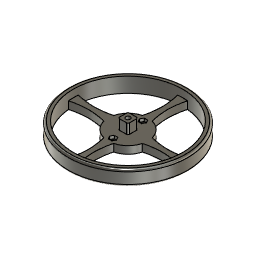
Balance v2 (Autodesk Fusion 360 design; units mm, degrees)
Autodesk Fusion 360 part; units mm, degrees
sketch "main" plane through (0, 0, 0) normal (0, 0, 1) x (1, 0, 0)
  circle A0 centre (0, 0) radius 2.25
  line L0 (-3.5, 5) -> (3.5, 5)
  line L1 (5, 3.5) -> (5, -3.5)
  line L2 (3.5, -5) -> (-3.5, -5)
  line L3 (-5, -3.5) -> (-5, 3.5)
  line L4 (-5, 5) -> (5, -5) construction
  line L5 (5, 5) -> (-5, -5) construction
  arc A1 (-3.5, 5) -> (-5, 3.5) centre (-3.5, 3.5) ccw
  arc A2 (-5, -3.5) -> (-3.5, -5) centre (-3.5, -3.5) ccw
  arc A3 (3.5, -5) -> (5, -3.5) centre (3.5, -3.5) ccw
  arc A4 (5, 3.5) -> (3.5, 5) centre (3.5, 3.5) ccw
  circle A5 centre (0, 0) radius 20
  line L6 (0, 5) -> (0, 15) construction
  line L7 (0, -15) -> (0, -5) construction
  circle A6 centre (0, 15) radius 1.75
  line L8 (3.465, 15) -> (1.7325, 18.0008)
  line L9 (1.7325, 18.0008) -> (-1.7325, 18.0008)
  line L10 (-1.7325, 18.0008) -> (-3.465, 15)
  line L11 (-3.465, 15) -> (-1.7325, 11.9992)
  line L12 (-1.7325, 11.9992) -> (1.7325, 11.9992)
  line L13 (1.7325, 11.9992) -> (3.465, 15)
  circle A7 centre (0, -15) radius 1.75
  line L14 (3.465, -15) -> (1.7325, -11.9992)
  line L15 (1.7325, -11.9992) -> (-1.7325, -11.9992)
  line L16 (-1.7325, -11.9992) -> (-3.465, -15)
  line L17 (-3.465, -15) -> (-1.7325, -18.0008)
  line L18 (-1.7325, -18.0008) -> (1.7325, -18.0008)
  line L19 (1.7325, -18.0008) -> (3.465, -15)
  circle A8 centre (0, 0) radius 55
  spline S0 degree 5 poles (-5.0305, 19.357) (-4.9656, 19.5382) (-4.8376, 19.914) (-4.6506, 20.5186) (-4.4115, 21.4066) (-4.1299, 22.6499) (-3.8662, 24.0155) (-3.6214, 25.4797) (-3.3969, 26.9998) (-3.1947, 28.5187) (-3.017, 29.9798) (-2.8658, 31.3385) (-2.7432, 32.5744) (-2.6507, 33.707) (-2.5895, 34.7948) (-2.5603, 35.9102) (-2.5641, 37.1227) (-2.6015, 38.476) (-2.6738, 39.9752) (-2.7821, 41.5999) (-2.9274, 43.3124) (-3.1108, 45.0674) (-3.3328, 46.8208) (-3.5937, 48.5404) (-3.8934, 50.2058) (-4.2314, 51.805) (-4.5322, 53.0272) (-4.7748, 53.9111) (-4.944, 54.4858) (-5.0305, 54.7695) knots 0 0 0 0 0 0 0.04 0.08 0.12 0.16 0.2 0.24 0.28 0.32 0.36 0.4 0.44 0.48 0.52 0.56 0.6 0.64 0.68 0.72 0.76 0.8 0.84 0.88 0.92 0.96 1 1 1 1 1 1
  spline S1 degree 5 poles (5.0305, 19.357) (4.9656, 19.5382) (4.8376, 19.914) (4.6506, 20.5186) (4.4115, 21.4066) (4.1299, 22.6499) (3.8662, 24.0155) (3.6214, 25.4797) (3.3969, 26.9998) (3.1947, 28.5187) (3.017, 29.9798) (2.8658, 31.3385) (2.7432, 32.5744) (2.6507, 33.707) (2.5895, 34.7948) (2.5603, 35.9102) (2.5641, 37.1227) (2.6015, 38.476) (2.6738, 39.9752) (2.7821, 41.5999) (2.9274, 43.3124) (3.1108, 45.0674) (3.3328, 46.8208) (3.5937, 48.5404) (3.8934, 50.2058) (4.2314, 51.805) (4.5322, 53.0272) (4.7748, 53.9111) (4.944, 54.4858) (5.0305, 54.7695) knots 0 0 0 0 0 0 0.04 0.08 0.12 0.16 0.2 0.24 0.28 0.32 0.36 0.4 0.44 0.48 0.52 0.56 0.6 0.64 0.68 0.72 0.76 0.8 0.84 0.88 0.92 0.96 1 1 1 1 1 1
  line L20 (-5.983, 16.697) -> (-4.078, 22.017)
  line L21 (-4.0792, 51.649) -> (-5.9817, 57.8899)
  line L22 (5.983, 16.697) -> (4.078, 22.017)
  line L23 (4.0792, 51.649) -> (5.9817, 57.8899)
  circle A9 centre (0, 0) radius 60
  point P0 (0, 15)
  point P1 (0, -15)
  point P2 (-3.7631, 24.6573)
  point P3 (-2.8027, 31.9975)
  point P4 (-2.5682, 36.8246)
  point P5 (-3.1758, 45.5337)
  point P6 (3.7631, 24.6573)
  point P7 (2.8027, 31.9975)
  point P8 (2.5682, 36.8246)
  point P9 (3.1758, 45.5337)
  dimension "d1" = 4.5
  dimension "d2" = 10
  dimension "d3" = 10
  dimension "d4" = 1.5
  dimension "d5" = 40
  dimension "d6" = 10
  dimension "d7" = 10
  dimension "d8" = 3.5
  dimension "d9" = 3.465
  dimension "d10" = 3.5
  dimension "d11" = 3.465
  dimension "d12" = 110
  dimension "d23" = 120
  constraint coincident A0.centre A5.centre
  constraint horizontal L0
  constraint perpendicular L0 L1
  constraint parallel L0 L2
  constraint parallel L1 L3
  constraint coincident L4 A0.centre
  constraint coincident L5 A0.centre
  constraint coincident L4.start L0
  constraint coincident L4.start L3
  constraint tangent L0 A1
  constraint tangent L3 A1
  constraint coincident L5.end L3
  constraint coincident L5.end L2
  constraint tangent L3 A2
  constraint tangent L2 A2
  constraint equal A1 A2
  constraint coincident L4.end L1
  constraint coincident L4.end L2
  constraint tangent L1 A3
  constraint tangent L2 A3
  constraint equal A1 A3
  constraint coincident L5.start L0
  constraint coincident L5.start L1
  constraint tangent L0 A4
  constraint tangent L1 A4
  constraint equal A1 A4
  constraint midpoint L0 L6.start
  constraint perpendicular L0 L6
  constraint coincident P0 L6.end
  constraint coincident P1 L7.start
  constraint coincident A5 S0.start
  constraint coincident A8 S0.end
  constraint midpoint S0.start L20
  constraint midpoint S0.end L21
  measures "d1" diameter of A0
  measures "d2" distance of L4.end L5.end
  measures "d3" distance of L5.start L4.end
  measures "d4" radius of A1
  measures "d5" diameter of A5
  measures "d6" distance of L6.start P0
  measures "d7" distance of P1 L7.end
  measures "d8" diameter of A6
  measures "d9" distance of L8.start P0
  measures "d10" diameter of A7
  measures "d11" distance of L14.start P1
  measures "d12" diameter of A8
  measures "d23" diameter of A9
extrude "Extrude1" add sketch "main" along normal blind 7.5 contours A5 A8 S0 S1 picked at (0.858, 27.2559) makes body 1
pattern_circular "C-Pattern1" count 4 over 360 about axis through (0, 0, 1.75) along (0, 0, 1) of "Extrude1" makes body 2 at (-23.1996, -4.0291, 2.7586) makes body 3 at (4.0291, -23.1996, 2.7586) makes body 4 at (23.1996, 4.0291, 2.7586)
extrude "Extrude2" add sketch "main" along normal blind 7.5 contours A5 bodies 1 2 3 4
extrude "Extrude3" add sketch "main" along normal blind 17.5 contours L0 L1 L2 L3 A1 A2 A3 A4 bodies 1
extrude "Extrude4" add sketch "main" along normal blind 4.5 contours L8 L9 L10 L11 L12 L13 | L14 L15 L16 L17 L18 L19 bodies 1
extrude "Extrude5" add sketch "main" along normal blind 15 contours A9 bodies 1
fillet "Fillet1" radius 2 2 edges at (-55.9396, -21.6969, 0) (-55.9396, -21.6969, 15) on bodies 1
equation "d9 = ( 6.93 / 2 ) * 1 mm"
equation "d11 = ( 6.93 / 2 ) * 1 mm"
equation "d21 = 7.50 mm - 3 mm"
named bodies: "Balance"
